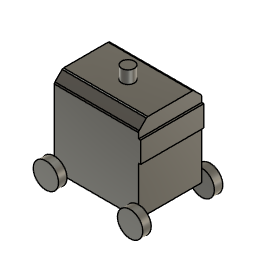
final v3 (Autodesk Fusion 360 design; units mm, degrees)
Autodesk Fusion 360 part; units mm, degrees
sketch "Sketch1" plane through (0, 0, 0) normal (0, 0, 1) x (1, 0, 0)
  line L0 (100, -75) -> (-100, -75)
  line L1 (-100, -75) -> (-100, 75)
  line L2 (-100, 75) -> (100, 75)
  line L3 (100, 75) -> (100, -75)
  line L4 (100, -75) -> (-100, 75) construction
  line L5 (-100, -75) -> (100, 75) construction
  dimension "d1" = 200
  dimension "d2" = 150
  constraint horizontal L0
  constraint perpendicular L0 L1
  constraint parallel L0 L2
  constraint parallel L1 L3
  constraint coincident L4 origin
  constraint coincident L5 origin
  measures "d1" distance of L1.end L2.end
  measures "d2" distance of L0.end L1.end
extrude "Extrude1" add sketch "Sketch1" along normal blind 200 makes body 1
sketch "Sketch2" plane through (0, -75, 0) normal (0, -1, 0) x (1, 0, 0)
  line L0 (-100, 0) -> (100, 0)
  line L1 (100, 0) -> (100, 200)
  line L2 (100, 200) -> (-100, 200)
  line L3 (-100, 200) -> (-100, 0)
move_body "Move1" bodies 1 to x (1, 0, 0) y (0, 1, 0) z (0, 0, 1) at (0, 0, 30)
sketch "Sketch3" plane through (0, -75, 0) normal (0, -1, 0) x (1, 0, 0)
  line L0 (-100, 30) -> (100, 30)
  line L1 (100, 30) -> (100, 230)
  line L2 (100, 230) -> (-100, 230)
  line L3 (-100, 230) -> (-100, 30)
  circle A0 centre (-100, 30) radius 30
  circle A1 centre (100, 30) radius 30
  constraint coincident L0.start L3.end
  constraint coincident L0.end L1.start
extrude "Extrude2" add sketch "Sketch3" along normal blind 20 separate body contours L0 L3 A0 | L0 L3 A0 makes body 2
extrude "Extrude3" add sketch "Sketch3" along normal blind 20 separate body contours L0 L1 A1 | L0 L1 A1 makes body 3
sketch "Sketch4" plane through (0, 75, 0) normal (0, 1, 0) x (-1, 0, 0)
  line L0 (-100, 30) -> (100, 30)
  line L1 (100, 30) -> (100, 230)
  line L2 (100, 230) -> (-100, 230)
  line L3 (-100, 230) -> (-100, 30)
  circle A0 centre (-100, 30) radius 30
  circle A1 centre (100, 30) radius 30
  constraint coincident L0.start L3.end
  constraint coincident L0.end L1.start
extrude "Extrude4" add sketch "Sketch4" along normal blind 20 separate body contours L0 L3 A0 | L0 L3 A0 | L0 L1 A1 | L0 L1 A1 makes body 4 at (70.1491, 81.6667, 27.013) makes body 5 at (-129.8509, 81.6667, 27.013)
sketch "Sketch5" plane through (0, 0, 230) normal (0, 0, 1) x (-1, 0, 0)
  line L0 (-100, -75) -> (100, -75)
  line L1 (100, -75) -> (100, 75)
  line L2 (100, 75) -> (-100, 75)
  line L3 (-100, 75) -> (-100, -75)
  circle A0 centre (0, 0) radius 15
  dimension "d11" = 30
  constraint coincident A0.centre origin
  measures "d11" diameter of A0
extrude "Extrude5" add sketch "Sketch5" along normal blind 30 contours A0 bodies 1
sketch "Sketch6" plane through (-100, 0, 0) normal (-1, 0, 0) x (0, -1, 0)
  line L0 (-75, 30) -> (75, 30)
  line L1 (75, 30) -> (75, 230)
  line L2 (75, 230) -> (-75, 230)
  line L3 (-75, 230) -> (-75, 30)
  line L4 (60, 160) -> (70, 160)
  line L5 (70, 160) -> (70, 140)
  line L6 (70, 140) -> (60, 140)
  line L7 (60, 140) -> (60, 160)
  constraint horizontal L4
  constraint vertical L5
  constraint horizontal L6
  constraint vertical L7
extrude "Extrude6" add sketch "Sketch6" along normal blind 5 contours L4 L5 L6 L7 bodies 1
sketch "Sketch7" plane through (100, 0, 0) normal (1, 0, 0) x (0, 1, 0)
  line L0 (-75, 30) -> (75, 30)
  line L1 (75, 30) -> (75, 230)
  line L2 (75, 230) -> (-75, 230)
  line L3 (-75, 230) -> (-75, 30)
  line L4 (85.2421, 145) -> (-85.2421, 145)
  line L5 (-85.2421, 145) -> (-85.2421, 195)
  line L6 (-85.2421, 195) -> (85.2421, 195)
  line L7 (85.2421, 195) -> (85.2421, 145)
  line L8 (85.2421, 145) -> (-85.2421, 195) construction
  line L9 (-85.2421, 145) -> (85.2421, 195) construction
  point P0 (0, 170)
  dimension "d16" = 50
  constraint horizontal L4
  constraint perpendicular L4 L5
  constraint parallel L4 L6
  constraint parallel L5 L7
  constraint coincident L8 P0
  constraint coincident L9 P0
  measures "d16" distance of L4.end L5.end
extrude "Extrude7" add sketch "Sketch7" along normal blind 5 contours L1 L3 L4 L6 bodies 1
delete_face "DeleteFace1" 1 faces at (-14.9255, 1.4935, 250) on bodies 1
sketch "Sketch8" plane through (0, 0, 230) normal (0, 0, 1) x (-1, 0, 0)
  line L0 (-100, -75) -> (100, -75)
  line L1 (100, -75) -> (100, 75)
  line L2 (100, 75) -> (-100, 75)
  line L3 (-100, 75) -> (-100, -75)
  circle A0 centre (0, 0) radius 15
  dimension "d19" = 30
  constraint coincident A0.centre origin
  measures "d19" diameter of A0
extrude "Extrude8" add sketch "Sketch8" along normal blind 30 separate body contours A0 makes body 6
chamfer "Chamfer1" distance 20 angle 45 2 edges at (0, 75, 230) (0, -75, 230) on bodies 1
fillet "Fillet1" radius 5 4 edges at (0, -75, 210) (0, -55, 230) (0, 55, 230) (0, 75, 210) on bodies 1
copy_body "Body->Comp1" bodies 1 removing the originals makes body 7 in component "base_link"
copy_body "Body->Comp2" bodies 2 removing the originals makes body 8 in component "rear_right_wheel"
copy_body "Body->Comp3" bodies 3 removing the originals makes body 9 in component "front_right_wheel"
copy_body "Body->Comp4" bodies 4 removing the originals makes body 10 in component "front_left_wheel"
copy_body "Body->Comp5" bodies 5 removing the originals makes body 11 in component "rear_left_wheel"
copy_body "Body->Comp6" bodies 6 removing the originals makes body 12 in component "lidar"
component "base_link" placed x (1, 0, 0) y (0, 1, 0) z (0, 0, 1) at (0, 0, 0)
component "rear_right_wheel" placed x (1, 0, 0) y (0, 1, 0) z (0, 0, 1) at (0, 0, 0)
component "front_right_wheel" placed x (1, 0, 0) y (0, 1, 0) z (0, 0, 1) at (0, 0, 0)
component "front_left_wheel" placed x (1, 0, 0) y (0, 1, 0) z (0, 0, 1) at (0, 0, 0)
component "rear_left_wheel" placed x (1, 0, 0) y (0, 1, 0) z (0, 0, 1) at (0, 0, 0)
component "lidar" placed x (1, 0, 0) y (0, 1, 0) z (0, 0, 1) at (0, 0, 0)
named bodies: "base_link", "rear_right_wheel", "front_right_wheel", "front_left_wheel", "rear_left_wheel", "lidar"
